Autodesk Fusion 360 part; units mm, degrees
note: some values were not read from the file. Set by a fixed rule: which sketch regions a step uses.
(part 4 of 4)
equation "d551 = 354.6390817817 * 0.5 mm"
equation "d552 = 354.6390817817 * 0.5 mm"
equation "d561 = 25.4 * 2 mm"
equation "d562 = 354.6390817817 * 0.5 mm"
equation "d563 = 354.6390817817 * 0.5 mm"
equation "d564 = 354.6390817817 * 0.5 mm"
equation "d565 = 354.6390817817 * 0.5 mm"
equation "d574 = 25.4 * 2 mm"
equation "d575 = 354.6390817817 * 0.5 mm"
equation "d576 = 354.6390817817 * 0.5 mm"
equation "d577 = 354.6390817817 * 0.5 mm"
equation "d578 = 354.6390817817 * 0.5 mm"
equation "d587 = 25.4 * 2 mm"
equation "d588 = 354.6390817817 * 0.5 mm"
equation "d589 = 354.6390817817 * 0.5 mm"
equation "d590 = 354.6390817817 * 0.5 mm"
equation "d591 = 354.6390817817 * 0.5 mm"
equation "d600 = 25.4 * 2 mm"
equation "d601 = 354.6390817817 * 0.5 mm"
equation "d602 = 354.6390817817 * 0.5 mm"
equation "d603 = 354.6390817817 * 0.5 mm"
equation "d604 = 354.6390817817 * 0.5 mm"
equation "d613 = 25.4 * 2 mm"
equation "d614 = 354.6390817817 * 0.5 mm"
equation "d615 = 354.6390817817 * 0.5 mm"
equation "d616 = 354.6390817817 * 0.5 mm"
equation "d617 = 354.6390817817 * 0.5 mm"
equation "d626 = 25.4 * 2 mm"
equation "d629 = 354.6390817817 * 0.5 mm"
equation "d630 = 354.6390817817 * 0.5 mm"
equation "d631 = 354.6390817817 * 0.5 mm"
equation "d632 = 354.6390817817 * 0.5 mm"
equation "d641 = 25.4 * 2 mm"
equation "d642 = 354.6390817817 * 0.5 mm"
equation "d643 = 354.6390817817 * 0.5 mm"
equation "d644 = 354.6390817817 * 0.5 mm"
equation "d645 = 354.6390817817 * 0.5 mm"
equation "d654 = 25.4 * 2 mm"
equation "d655 = 354.6390817817 * 0.5 mm"
equation "d656 = 354.6390817817 * 0.5 mm"
equation "d657 = 354.6390817817 * 0.5 mm"
equation "d658 = 354.6390817817 * 0.5 mm"
equation "d667 = 25.4 * 2 mm"
equation "d668 = 354.6390817817 * 0.5 mm"
equation "d669 = 354.6390817817 * 0.5 mm"
equation "d670 = 354.6390817817 * 0.5 mm"
equation "d671 = 354.6390817817 * 0.5 mm"
equation "d680 = 25.4 * 2 mm"
equation "d681 = 354.6390817817 * 0.5 mm"
equation "d682 = 354.6390817817 * 0.5 mm"
equation "d683 = 354.6390817817 * 0.5 mm"
equation "d684 = 354.6390817817 * 0.5 mm"
equation "d693 = 25.4 * 2 mm"
equation "d697 = 354.6390817817 * 0.5 mm"
equation "d698 = 354.6390817817 * 0.5 mm"
equation "d699 = 354.6390817817 * 0.5 mm"
equation "d700 = 354.6390817817 * 0.5 mm"
equation "d709 = 25.4 * 2 mm"
equation "d710 = 354.6390817817 * 0.5 mm"
equation "d711 = 354.6390817817 * 0.5 mm"
equation "d712 = 354.6390817817 * 0.5 mm"
equation "d713 = 354.6390817817 * 0.5 mm"
equation "d722 = 25.4 * 2 mm"
equation "d723 = 354.6390817817 * 0.5 mm"
equation "d724 = 354.6390817817 * 0.5 mm"
equation "d725 = 354.6390817817 * 0.5 mm"
equation "d726 = 354.6390817817 * 0.5 mm"
equation "d735 = 25.4 * 2 mm"
equation "d737 = 354.6390817817 * 0.5 mm"
equation "d738 = 354.6390817817 * 0.5 mm"
equation "d739 = 354.6390817817 * 0.5 mm"
equation "d740 = 354.6390817817 * 0.5 mm"
equation "d749 = 25.4 * 2 mm"
equation "d750 = 354.6390817817 * 0.5 mm"
equation "d751 = 354.6390817817 * 0.5 mm"
equation "d752 = 354.6390817817 * 0.5 mm"
equation "d753 = 354.6390817817 * 0.5 mm"
equation "d762 = 25.4 * 2 mm"
equation "d763 = 354.6390817817 * 0.5 mm"
equation "d764 = 354.6390817817 * 0.5 mm"
equation "d765 = 354.6390817817 * 0.5 mm"
equation "d766 = 354.6390817817 * 0.5 mm"
equation "d775 = 25.4 * 2 mm"
equation "d776 = 354.6390817817 * 0.5 mm"
equation "d777 = 354.6390817817 * 0.5 mm"
equation "d778 = 354.6390817817 * 0.5 mm"
equation "d779 = 354.6390817817 * 0.5 mm"
equation "d788 = 25.4 * 2 mm"
equation "d789 = 354.6390817817 * 0.5 mm"
equation "d790 = 354.6390817817 * 0.5 mm"
equation "d791 = 354.6390817817 * 0.5 mm"
equation "d792 = 354.6390817817 * 0.5 mm"
equation "d801 = 25.4 * 2 mm"
equation "d802 = 354.6390817817 * 0.5 mm"
equation "d803 = 354.6390817817 * 0.5 mm"
equation "d804 = 354.6390817817 * 0.5 mm"
equation "d805 = 354.6390817817 * 0.5 mm"
equation "d814 = 25.4 * 2 mm"
equation "d815 = 354.6390817817 * 0.5 mm"
equation "d816 = 354.6390817817 * 0.5 mm"
equation "d817 = 354.6390817817 * 0.5 mm"
equation "d818 = 354.6390817817 * 0.5 mm"
equation "d827 = 25.4 * 2 mm"
equation "d828 = 354.6390817817 * 0.5 mm"
equation "d829 = 354.6390817817 * 0.5 mm"
equation "d830 = 354.6390817817 * 0.5 mm"
equation "d831 = 354.6390817817 * 0.5 mm"
equation "d840 = 25.4 * 2 mm"
equation "d841 = 354.6390817817 * 0.5 mm"
equation "d842 = 354.6390817817 * 0.5 mm"
equation "d843 = 354.6390817817 * 0.5 mm"
equation "d844 = 354.6390817817 * 0.5 mm"
equation "d853 = 25.4 * 2 mm"
equation "d854 = 354.6390817817 * 0.5 mm"
equation "d855 = 354.6390817817 * 0.5 mm"
equation "d856 = 354.6390817817 * 0.5 mm"
equation "d857 = 354.6390817817 * 0.5 mm"
equation "d866 = 25.4 * 2 mm"
equation "d867 = 354.6390817817 * 0.5 mm"
equation "d868 = 354.6390817817 * 0.5 mm"
equation "d869 = 354.6390817817 * 0.5 mm"
equation "d870 = 354.6390817817 * 0.5 mm"
equation "d879 = 25.4 * 2 mm"
equation "d880 = 354.6390817817 * 0.5 mm"
equation "d881 = 354.6390817817 * 0.5 mm"
equation "d882 = 354.6390817817 * 0.5 mm"
equation "d883 = 354.6390817817 * 0.5 mm"
equation "d892 = 25.4 * 2 mm"
equation "d893 = 354.6390817817 * 0.5 mm"
equation "d894 = 354.6390817817 * 0.5 mm"
equation "d895 = 354.6390817817 * 0.5 mm"
equation "d896 = 354.6390817817 * 0.5 mm"
equation "d918 = 25.4 * 2 mm"
equation "d921 = 354.6390817817 * 0.5 mm"
equation "d922 = 354.6390817817 * 0.5 mm"
equation "d924 = 354.6390817817 * 0.5 mm"
equation "d925 = 354.6390817817 * 0.5 mm"
equation "d940 = 25.4 * 2 mm"
equation "d944 = 354.6390817817 * 0.5 mm"
equation "d945 = 354.6390817817 * 0.5 mm"
equation "d946 = 354.6390817817 * 0.5 mm"
equation "d947 = 354.6390817817 * 0.5 mm"
equation "d958 = 25.4 * 2 mm"
equation "d959 = 354.6390817817 * 0.5 mm"
equation "d960 = 354.6390817817 * 0.5 mm"
equation "d961 = 354.6390817817 * 0.5 mm"
equation "d962 = 354.6390817817 * 0.5 mm"
equation "d971 = 25.4 * 2 mm"
equation "d975 = 70.00 mm + 15 mm + 20 mm"
